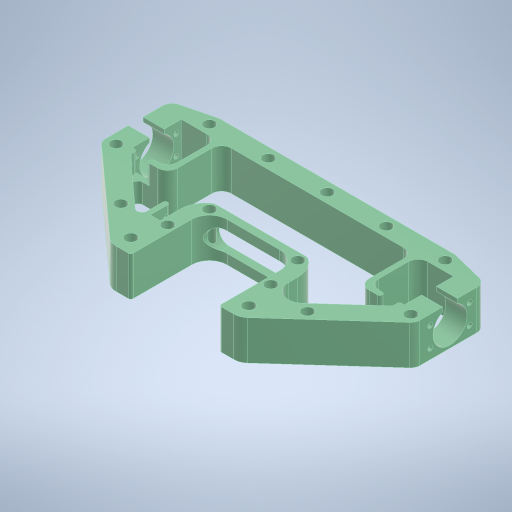
# Autodesk Inventor part: Chassis
Saved by Autodesk Inventor 2023.1 (Build 271208000, 208)
## iProperties
Created: 2022-05-26
Part Number: Chassis
Material: Nylon 6/6
Document SubType Name: Modeling
Designer: Nathan Cai
Density: 0.860238 g/cm^3
Appearance: Smooth - Dark Sea Green
Mass: 136 g
Surface Area: 542.617 cm^2
Volume: 158.096 cm^3
Author: Nathan Cai
Autodesk Inventor part; units mm, degrees
ref_plane "YZ Plane" through (0, 0, 0) normal (1, 0, 0) x (0, 1, 0)
ref_plane "XZ Plane" through (0, 0, 0) normal (0, 1, 0) x (-1, 0, 0)
ref_plane "XY Plane" through (0, 0, 0) normal (0, 0, 1) x (1, 0, 0)
sketch "Sketch1" plane through (0, 0, 0) normal (0, 1, 0) x (-1, 0, 0)
  line L0 (101.6, 38.1) -> (-101.6, 38.1) construction
  line L1 (-101.6, 38.1) -> (-101.6, -38.1) construction
  line L2 (-101.6, -38.1) -> (101.6, -38.1)
  line L3 (101.6, -38.1) -> (101.6, 38.1) construction
  line L4 (101.6, 38.1) -> (-101.6, -38.1) construction
  line L5 (-101.6, 38.1) -> (101.6, -38.1) construction
  line L6 (-28.575, 66.675) -> (28.575, 66.675) construction
  line L7 (28.575, 66.675) -> (28.575, 9.525)
  line L8 (28.575, 9.525) -> (-28.575, 9.525)
  line L9 (-28.575, 9.525) -> (-28.575, 66.675)
  line L10 (-28.575, 66.675) -> (28.575, 9.525) construction
  line L11 (28.575, 66.675) -> (-28.575, 9.525) construction
  circle A0 centre (-38.1, 50.8) radius 3.556
  line L12 (0, 38.1) -> (0, -38.1) construction
  circle A1 centre (-38.1, 50.8) radius 9.525
  line L13 (-38.1, 60.325) -> (-28.575, 60.325)
  circle A2 centre (38.1, 50.8) radius 3.556
  circle A3 centre (38.1, 50.8) radius 9.525
  line L14 (38.1, 60.325) -> (28.575, 60.325)
  circle A4 centre (-76.2, -38.1) radius 3.4925
  circle A5 centre (-95.25, 3.175) radius 3.4925
  circle A6 centre (76.2, -38.1) radius 3.4925
  circle A7 centre (95.25, 3.175) radius 3.4925
  line L15 (-101.6, -38.1) -> (-101.6, 6.35)
  line L16 (-101.6, 6.35) -> (-44.479723, 57.872818)
  line L17 (101.6, -38.1) -> (101.6, 6.35)
  line L18 (101.6, 6.35) -> (44.479723, 57.872818)
  line L19 (-42.641743, 42.427533) -> (-87.975, 1.536675)
  line L20 (-87.975, 1.536675) -> (-87.975, -38.1)
  line L21 (87.975, -38.1) -> (87.975, 1.536675)
  line L22 (87.975, 1.536675) -> (42.641743, 42.427533)
  line L23 (0, -38.1) -> (-95.25, -38.1)
  line L24 (0, -38.1) -> (95.25, -38.1) construction
  circle A8 centre (-60.325, 35.028711) radius 3.4925
  circle A9 centre (-33.3375, 31.75) radius 3.4925
  line L25 (-38.1, 0) -> (-38.1, 41.275)
  line L26 (-38.1, 0) -> (0, 0) construction
  circle A10 centre (60.325, 35.028711) radius 3.4925
  circle A11 centre (33.3375, 31.75) radius 3.4925
  line L27 (38.1, 0) -> (38.1, 41.275)
  line L28 (38.1, 0) -> (0, 0) construction
  line L29 (-87.975, 0) -> (-65.115, 0)
  line L30 (-65.115, 0) -> (-65.115, -31.75)
  line L31 (-65.115, -31.75) -> (-87.975, -31.75)
  line L32 (-101.6, -38.1) -> (101.6, -38.1) construction
  line L33 (101.6, -38.1) -> (101.6, 19.05)
  line L34 (101.6, 19.05) -> (-101.6, 19.05) construction
  line L35 (-101.6, 19.05) -> (-101.6, -38.1)
  line L36 (-101.6, 19.05) -> (-87.520267, 19.05) construction
  line L37 (87.520267, 19.05) -> (101.6, 19.05) construction
  circle A12 centre (-38.1, 0) radius 3.175 construction
  circle A13 centre (-38.1, 0) radius 6.35 construction
  circle A14 centre (38.1, 0) radius 3.175 construction
  circle A15 centre (38.1, 0) radius 6.35 construction
  circle A16 centre (28.575, 9.525) radius 3.4925
  circle A17 centre (28.575, 9.525) radius 4.7625
  arc A18 (17.077308, 9.525) -> (28.575, 21.022692) centre (17.077308, 21.022692) ccw
  circle A19 centre (-28.575, 9.525) radius 3.4925
  circle A20 centre (-28.575, 9.525) radius 4.7625
  arc A21 (-28.575, 21.022692) -> (-17.077308, 9.525) centre (-17.077308, 21.022692) ccw
  arc A22 (31.4325, 5.715) -> (38.1, 19.05) centre (21.43125, 19.05) ccw
  arc A23 (-38.1, 19.05) -> (-31.4325, 5.715) centre (-21.43125, 19.05) ccw
  line L38 (-61.94, -38.1) -> (-61.94, 25.020395)
  line L39 (87.975, 0) -> (65.115, 0)
  line L40 (65.115, 0) -> (65.115, -31.75)
  line L41 (65.115, -31.75) -> (87.975, -31.75)
  line L42 (61.94, -38.1) -> (61.94, 25.020395)
  line L43 (-28.575, 4.7625) -> (28.575, 4.7625)
  line L44 (101.6, -31.75) -> (-101.6, -31.75)
  line L45 (-101.6, -31.75) -> (-101.6, -44.45) construction
  line L46 (-101.6, -44.45) -> (101.6, -44.45)
  line L47 (101.6, -44.45) -> (101.6, -31.75) construction
  circle A24 centre (0, -38.1) radius 3.4925
  circle A25 centre (38.1, -38.1) radius 3.4925
  circle A26 centre (-38.1, -38.1) radius 3.4925
  line L48 (101.6, -38.1) -> (76.2, -44.45)
  line L49 (-101.6, -38.1) -> (-76.2, -44.45)
  line L50 (76.2, -38.1) -> (76.2, -44.45) construction
  line L51 (-76.2, -38.1) -> (-76.2, -44.45) construction
  line L52 (-61.94, 3.175) -> (-86.158686, 3.175)
  line L53 (61.94, 3.175) -> (86.158686, 3.175)
  line L54 (38.1, 19.05) -> (44.45, 19.05)
  line L55 (44.45, 19.05) -> (44.45, 31.75)
  line L56 (44.45, 31.75) -> (38.1, 31.75)
  line L57 (38.1, 31.75) -> (38.1, 19.05)
  line L58 (38.1, 19.05) -> (47.625, 19.05)
  line L59 (47.625, 19.05) -> (47.625, 37.932607)
  line L60 (47.625, 37.932607) -> (38.1, 37.932607) construction
  line L61 (38.1, 37.932607) -> (38.1, 19.05)
  point P0 (28.575, 38.1)
  point P1 (-28.575, 38.1)
  point P2 (28.575, 60.325)
  point P3 (44.479723, 57.872818)
  point P4 (101.6, -15.875)
  point P5 (38.1, 41.275)
  point P6 (-87.975, -31.75)
  point P7 (-101.6, 6.35)
  point P8 (101.6, 6.35)
  point P9 (31.75, 0)
  point P10 (38.1, 6.35)
  point P11 (-38.1, 6.35)
  point P12 (-31.75, 0)
  point P13 (87.975, 0)
  point P14 (61.94, 25.020395)
  point P15 (-17.077308, 9.525)
  point P16 (-28.575, 21.022692)
  point P17 (-38.1, 19.05)
  point P18 (-31.4325, 5.715)
  point P19 (-21.850242, 0)
  point P20 (21.850242, 0)
  point P21 (-25.207404, 12.892596)
  point P22 (-28.575, 14.2875)
  point P23 (-23.8125, 9.525)
  point P24 (-28.575, 50.8)
  point P25 (25.207404, 12.892596)
  point P26 (28.575, 14.2875)
  point P27 (23.8125, 9.525)
  point P28 (28.575, 50.8)
  point P29 (25.0825, 9.525)
  point P30 (28.575, 13.0175)
  point P31 (61.94, -31.75)
  point P32 (-61.94, -31.75)
  dimension "d0" = 203.2
  dimension "d1" = 76.2
  dimension "d4" = 57.15
  dimension "d6" = 7.112
  dimension "d7" = 38.1
  dimension "d8" = 19.05
  dimension "d10" = 6.985
  dimension "d11" = 6.985
  dimension "d12" = 0
  dimension "d14" = 25.4
  dimension "d15" = 6.35
  dimension "d20" = 50.8
  dimension "d21" = 41.275
  dimension "d22" = 44.45
  dimension "d24" = 12.7
  dimension "d25" = 13.625
  dimension "d26" = 12.7
  dimension "d27" = 13.625
  dimension "d31" = 6.985
  dimension "d32" = 6.985
  dimension "d33" = 6.35
  dimension "d34" = 31.75
  dimension "d35" = 4.7625
  dimension "d36" = 22.225
  dimension "d37" = 9.525
  dimension "d39" = 31.75
  dimension "d40" = 6.35
  dimension "d42" = 57.15
  dimension "d43" = 6.35
  dimension "d44" = 9.525
  dimension "d45" = 9.525
  dimension "d46" = 12.7
  dimension "d104" = 6.985
  dimension "d105" = 9.525
  dimension "d106" = 3.175
  dimension "d107" = 22.86
  dimension "d123" = 88.9
  dimension "d124" = 12.7
  dimension "d125" = 6.985
  dimension "d126" = 6.985
  dimension "d127" = 38.1
  dimension "d128" = 28.575
  dimension "d134" = 3.175
  dimension "d137" = 6.35
  dimension "d138" = 12.7
  dimension "d139" = 9.525
  constraints: 125 end point, 32 symmetric about line, 26 centre point, 25 point on line, 16 parallel, 16 point on circle, 11 horizontal, 9 perpendicular, 8 midpoint, 8 tangent, 7 coincident, 2 vertical, 1 collinear, 16 other
  measures "d0" distance of L2.end L1.end
  measures "d1" distance between parallel lines of L0 L2
  measures "d4" distance of L7.end L8.end
  measures "d6" diameter of A0
  measures "d7" distance from line of L12 A0.centre
  measures "d8" diameter of A1
  measures "d10" diameter of A4
  measures "d11" diameter of A5
  measures "d12" distance from line of L2 L51.start
  measures "d14" distance from line of L1 L51.start
  measures "d15" distance from line of L1 A5.centre
  measures "d20" distance between parallel lines of L8 L14
  measures "d21" vertical distance of L51.start A5.centre
  measures "d22" distance of L1.end L15.end
  measures "d24" distance between parallel lines of L16 L19
  measures "d25" distance between parallel lines of L15 L20
  measures "d26" distance between parallel lines of L18 L22
  measures "d27" distance from line of point (101.6, -15.875) L21
  measures "d31" diameter of A8
  measures "d32" diameter of A9
  measures "d33" distance from line of L16 A8.centre
  measures "d34" distance from line of L9 A8.centre
  measures "d35" distance from line of L9 A9.centre
  measures "d36" distance from line of L8 A9.centre
  measures "d37" distance between parallel lines of L9 L25
  measures "d39" distance between parallel lines of L31 L29
  measures "d40" distance between parallel lines of L23 L31
  measures "d42" distance of L33.end L32.end
  measures "d43" diameter of A12
  measures "d44" distance from line of L8 A12.centre
  measures "d45" distance from line of L9 A12.centre
  measures "d46" diameter of A13
  measures "d104" diameter of A16
  measures "d105" diameter of A17
  measures "d106" distance between parallel lines of L30 L38
  measures "d107" distance between parallel lines of L20 L30
  measures "d123" distance from line of L32 A1.centre
  measures "d124" distance between parallel lines of L44 L46
  measures "d125" diameter of A24
  measures "d126" diameter of A25
  measures "d127" distance of A24.centre A25.centre
  measures "d128" distance from line of L12 A16.centre
  measures "d134" distance between parallel lines of L29 L52
  measures "d137" distance of L56.end L55.end
  measures "d138" distance of L55.end L54.end
  measures "d139" distance of L60.end L59.end
extrude "Extrusion1" add sketch "Sketch1" along normal blind 25.4 contours L15 L44 L20 L2 | L2 A4 A26 A24 A25 A6 L48 L46 L49 | L15 L16 A1 L19 L20 L44 | L20 L31 L44 L38 L2 A4 | A1 | L20 L19 L52 L38 L44 L30 L29 | L2 L21 L44 L17 | L13 L9 A1 | L44 L42 L2 A25 A24 A26 L38 | L2 A6 L42 L44 L41 L21 | L44 L21 L22 A3 L18 L17 | L9 A20 A23 L25 A1 | L42 L53 L22 L21 L39 L40 L44 | A21 A20 L9 | A3 | A20 L8 A19 L9 | L9 A19 L8 A20 | A21 L8 A20 | A3 L7 L14 | L8 A17 L43 A20 | L59 L58 L55 L56 L27 A3 L22 | A3 L27 A22 A17 L7 | A18 A17 L8 | A17 L8 A16 L7 | L7 A17 A18 | A17 L7 A16 L8 | L54 L27 L56 L55
fillet "Fillet1" radius 6.35 14 edges at (65.115, 12.7, 0) (65.115, 12.7, -31.75) (101.6, 12.7, -38.1) (101.6, 12.7, 6.35) (-101.6, 12.7, 6.35) (-65.115, 12.7, -31.75) (-65.115, 12.7, 0) (-61.94, 12.7, -31.75) (61.94, 12.7, -31.75) (76.2, 12.7, -44.45) (-76.2, 12.7, -44.45) (-101.6, 12.7, -38.1) (61.94, 12.7, 3.175) (-61.94, 12.7, 3.175)
sketch "Sketch2" plane through (0, 25.4, 0) normal (0, 1, 0) x (1, 0, 0)
  line L0 (-38.1, -19.05) -> (-47.625, -19.05) projected
  line L1 (-38.1, -19.05) -> (-44.45, -19.05)
  line L2 (-44.45, -19.05) -> (-44.45, -31.75)
  line L3 (-44.45, -31.75) -> (-38.1, -31.75)
  line L4 (-38.1, -31.75) -> (-38.1, -19.05)
  point P0 (0, 0)
  dimension "d140" = 6.35
  dimension "d141" = 12.7
  constraints: 8 end point, 2 parallel, 1 horizontal, 1 perpendicular
  measures "d140" distance of L3.end L2.end
  measures "d141" distance of L2.end L1.end
extrude "Extrusion2" cut sketch "Sketch2" against normal blind 12.7
fillet "Fillet2" radius 3.175 2 edges at (-86.1587, 12.7, 3.175) (86.1587, 12.7, 3.175)
sketch "Sketch3" plane through (101.6, 0, 15.875) normal (1, 0, 0) x (0, 0, -1)
  circle A0 centre (31.75, 12.7) radius 11
  line L0 (0, 25.4) -> (50.8, 25.4) projected
  line L1 (50.8, 0) -> (50.8, 25.4) projected
  circle A1 centre (19.05, 6.35) radius 1.5875
  line L2 (0, 0) -> (50.8, 0) projected
  circle A2 centre (44.45, 6.35) radius 1.5875
  circle A3 centre (19.05, 19.05) radius 1.5875
  circle A4 centre (44.45, 19.05) radius 1.5875
  point P0 (15.875, 0)
  dimension "d54" = 22
  dimension "d55" = 12.7
  dimension "d56" = 19.05
  dimension "d63" = 3.175
  dimension "d64" = 6.35
  dimension "d65" = 12.7
  dimension "d68" = 25.4
  dimension "d71" = 12.7
  constraints: 5 centre point, 1 horizontal, 1 vertical, 6 other
  measures "d54" diameter of A0
  measures "d55" distance from line of L0 A0.centre
  measures "d56" distance from line of L1 A0.centre
  measures "d63" diameter of A1
  measures "d64" distance from line of L2 A1.centre
  measures "d65" horizontal distance of A0.centre A1.centre
  measures "d68" distance of A1.centre A2.centre
  measures "d71" distance of A1.centre A3.centre
extrude "Extrusion3" cut sketch "Sketch3" against normal blind 19.05
sketch "Sketch4" plane through (0, 25.4, 0) normal (0, 1, 0) x (1, 0, 0)
  line L0 (101.6, 11.1125) -> (87.975, 11.1125)
  line L1 (87.975, 11.1125) -> (87.975, 20.6375)
  line L2 (87.975, 20.6375) -> (101.6, 20.6375)
  line L3 (101.6, 20.6375) -> (101.6, 11.1125)
  line L4 (44.45, 47.625) -> (-44.45, 47.625)
  line L5 (71.465, 31.75) -> (87.975, 31.75)
  line L6 (87.975, 0) -> (71.465, 0)
  line L7 (61.94, 25.4) -> (61.94, 3.175)
  line L8 (87.975, 0) -> (61.94, 0)
  line L9 (61.94, 0) -> (61.94, -12.7)
  line L10 (61.94, -12.7) -> (87.975, -12.7)
  line L11 (87.975, -12.7) -> (87.975, 0) construction
  line L12 (87.975, -12.7) -> (84.8, -12.7)
  line L13 (84.8, -12.7) -> (84.8, 0)
  line L14 (84.8, 0) -> (87.975, 0)
  line L15 (87.975, 0) -> (87.975, -12.7) construction
  line L16 (80.025016, -8.707606) -> (42.641743, -42.427533)
  line L17 (75.598887, -12.7) -> (84.8, -4.400543)
  line L18 (75.275, 0) -> (75.275, -12.7)
  point P0 (0, 0)
  point P1 (88.9, 47.625)
  point P2 (-88.9, 47.625)
  point P3 (101.6, 33.14207)
  point P4 (61.94, 31.75)
  point P5 (61.94, -22.196554)
  point P6 (84.8, 0)
  point P7 (61.94, 0)
  point P8 (61.94, -3.175)
  dimension "d59" = 9.525
  dimension "d60" = 26.9875
  dimension "d112" = 12.7
  dimension "d113" = 3.175
  dimension "d135" = 9.525
  constraints: 28 end point, 9 point on line, 6 parallel, 4 perpendicular, 3 horizontal, 1 collinear
  measures "d59" distance of L0.end L1.end
  measures "d60" distance between parallel lines of L4 L2
  measures "d112" distance of L9.end L8.end
  measures "d113" distance of L13.end L14.end
  measures "d135" distance between parallel lines of L13 L18
extrude "Extrusion4" cut sketch "Sketch4" against normal blind 12.7 contours L0 L1 L2 L3 | L13 L17 L16 L10 L18 L6
ref_plane "Work Plane1" through (0, 0, 53.975) normal (1, 0, 0) x (0, 0, -1)
mirror "Mirror1" about plane through (0, 0, 53.975) normal (1, 0, 0) of "Extrusion3", "Extrusion4"
fillet "Fillet3" radius 1.5875 10 edges at (84.8, 19.05, 0) (-84.8, 19.05, 0) (84.8, 19.05, 4.4005) (75.275, 19.05, 3.175) (75.275, 19.05, 0) (-84.8, 19.05, 4.4005) (-44.45, 19.05, 19.05) (-47.625, 12.7, 19.05) (-75.275, 19.05, 0) (-75.275, 19.05, 3.175)
sketch "Sketch6" plane through (-22.225, 0, 9.525) normal (0, 0, 1) x (1, 0, 0)
  line L0 (5.147692, 25.4) -> (39.302308, 25.4)
  line L1 (22.225, 25.4) -> (22.225, 0) construction
  line L2 (1.5875, 12.7) -> (42.8625, 12.7) construction
  line L3 (1.5875, 6.35) -> (42.8625, 6.35)
  line L4 (42.8625, 19.05) -> (1.5875, 19.05)
  arc A0 (1.5875, 19.05) -> (1.5875, 6.35) centre (1.5875, 12.7) ccw
  arc A1 (42.8625, 6.35) -> (42.8625, 19.05) centre (42.8625, 12.7) ccw
  line L5 (17.4625, 6.35) -> (26.9875, 6.35)
  line L6 (26.9875, 6.35) -> (26.9875, 19.05)
  line L7 (26.9875, 19.05) -> (17.4625, 19.05)
  line L8 (17.4625, 19.05) -> (17.4625, 6.35)
  line L9 (17.4625, 6.35) -> (26.9875, 19.05) construction
  line L10 (26.9875, 6.35) -> (17.4625, 19.05) construction
  point P0 (0, 25.4)
  point P1 (44.45, 25.4)
  point P2 (22.225, 12.7)
  point P3 (-6.35, 25.4)
  point P4 (50.8, 25.4)
  point P5 (1.5875, 25.4)
  dimension "d92" = 20.6375
  dimension "d93" = 12.7
  dimension "d136" = 9.525
  constraints: 22 end point, 5 midpoint, 4 point on circle, 4 tangent, 3 parallel, 2 centre point, 2 perpendicular, 1 horizontal, 1 point on line, 1 vertical
  measures "d92" distance of point (22.225, 12.7) L2.end
  measures "d93" diameter of A1
  measures "d136" distance of L7.end L6.end
extrude "Extrusion6" cut sketch "Sketch6" along normal mid plane 25.4
fillet "Fillet4" radius 9.525 2 edges at (38.1, 12.7, 41.275) (42.6417, 12.7, 42.4275)
fillet "Fillet5" radius 1.5875 2 edges at (-28.575, 12.7, 60.325) (28.575, 12.7, 60.325)
fillet "Fillet6" radius 3.175 1 edges at (-47.625, 12.7, 37.9326)
sketch "Sketch8" plane through (-47.625, 0, 20.6375) normal (-1, 0, 0) x (0, 0, 1)
  point P0 (0.9525, 19.05)
  point P1 (8.5725, 19.05)
hole "Hole2" at (-47.625, 19.05, 21.59) at (-47.625, 19.05, 29.21) direction (1, 0, 0) diameter 2.4384 depth 3.175
equation "\"d35\" = 0.5 * d37"
body "Solid1"
